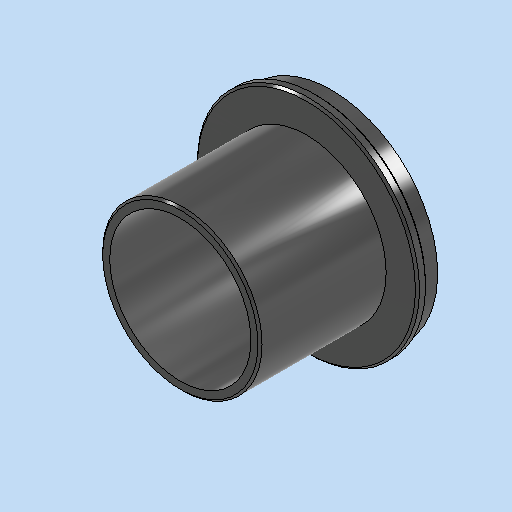
# Autodesk Inventor part: M42-nose-peace
Saved by Autodesk Inventor 2025 (Build 290162000, 162)
## iProperties
Created: 2025-02-20
Part Number: M42-nose-peace
Material: Aluminum 6061
Document SubType Name: Modeling
Designer: kuzmin
Density: 2.7 g/cm^3
Appearance: Dark Gray
Author: kuzmin
Autodesk Inventor part; units mm, degrees
ref_plane "YZ Plane" through (0, 0, 0) normal (1, 0, 0) x (0, 1, 0)
ref_plane "XZ Plane" through (0, 0, 0) normal (0, 1, 0) x (-1, 0, 0)
ref_plane "XY Plane" through (0, 0, 0) normal (0, 0, 1) x (1, 0, 0)
sketch "Sketch1" plane through (0, 0, 0) normal (0, 1, 0) x (-1, 0, 0)
  line L0 (0, 0) -> (0, 30)
  line L1 (15.8, 30) -> (15.8, 5)
  line L2 (15.8, 5) -> (22, 5)
  line L3 (22, 5) -> (22, 3)
  line L4 (22, 3) -> (21, 3)
  line L5 (21, 3) -> (21, 0)
  line L6 (0, 30) -> (14, 30) construction
  line L7 (14, 30) -> (15.8, 30)
  line L8 (21, 0) -> (14, 0)
  line L9 (14, 0) -> (0, 0) construction
  line L10 (14, 30) -> (14, 0)
  dimension "d0" = 28
  dimension "d1" = 31.6
  dimension "d2" = 44
  dimension "d3" = 42
  dimension "d4" = 3
  dimension "d5" = 2
  dimension "d6" = 25
  constraints: 22 end point, 4 perpendicular, 2 collinear, 2 horizontal, 2 vertical
  measures "d0" diameter of L10 L0
  measures "d1" diameter of L1 L0
  measures "d2" diameter of L3 L0
  measures "d3" diameter of L5 L0
  measures "d4" distance of L4.end L5.end
  measures "d5" distance of L2.end L3.end
  measures "d6" distance of L1.start L1.end
revolve "Revolution1" add sketch "Sketch1" angle 360 about axis through (0, 0, 0) along (0, 0, 1)
chamfer "Chamfer1" distance 0.4 angle 45 3 edges at (15.8, 0, 30) (22, 0, 5) (22, 0, 3)
body "Solid1"
